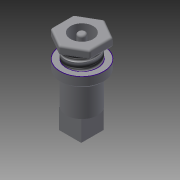
# Autodesk Inventor part: Power_Socket
Saved by Autodesk Inventor 2015 (Build 190159000, 159)
## iProperties
Created: 2014-12-09
Part Number: Power_Socket
Material: Generic
Document SubType Name: Modeling
Designer: Temp2
Density: 1 g/cm^3
Appearance: Default
Author: Temp2
Autodesk Inventor part; units mm, degrees
ref_plane "YZ Plane" through (0, 0, 0) normal (1, 0, 0) x (0, 1, 0)
ref_plane "XZ Plane" through (0, 0, 0) normal (0, 1, 0) x (-1, 0, 0)
ref_plane "XY Plane" through (0, 0, 0) normal (0, 0, 1) x (1, 0, 0)
sketch "Sketch1" plane through (0, 0, 0) normal (0, 0, 1) x (1, 0, 0)
  circle A0 centre (0, 0) radius 5.5
  circle A1 centre (0, 0) radius 1
  circle A2 centre (0, 0) radius 3.9688
  circle A3 centre (0, 0) radius 2.85
  dimension "d0" = 11
  dimension "d1" = 2
  dimension "d2" = 7.9375
  dimension "d3" = 5.7
  constraints: 4 centre point, 4 coincident
  measures "d0" diameter of A0
  measures "d1" diameter of A1
  measures "d2" diameter of A2
  measures "d3" diameter of A3
extrude "Extrusion1" add sketch "Sketch1" along normal blind 5.7 and the other way blind 10.4 contours A2
extrude "Extrusion2" add sketch "Sketch1" against normal blind 2.7 contours A0
extrude "Extrusion3" add sketch "Sketch1" along normal blind 5.7 contours A1
extrude "Extrusion4" add sketch "Sketch1" against normal blind 2.7 contours A1 | A2 | A3
sketch "Sketch2" plane through (0, 0, -10.4) normal (0, 0, -1) x (-1, 0, 0)
  circle A0 centre (0, 0) radius 3.9688 projected
  line L0 (2.8725, 2.7386) -> (-2.7241, 2.7386)
  line L1 (-2.7241, 2.7386) -> (-2.7241, -2.8862)
  line L2 (-2.7241, -2.8862) -> (2.8725, -2.8862)
  line L3 (2.8725, -2.8862) -> (2.8725, 2.7386)
  constraints: 8 end point, 2 parallel, 2 point on circle, 1 horizontal, 1 perpendicular
extrude "Extrusion5" add sketch "Sketch2" along normal blind 5.2 contours L3 A0 L2 L1 L0 | L3 L2 A0
sketch "Sketch3" plane through (0, 0, 5.7) normal (0, 0, 1) x (1, 0, 0)
  line L0 (5, -2.8868) -> (5, 2.8868)
  line L1 (0, 5.7735) -> (5, 2.8868)
  line L2 (0, 5.7735) -> (-5, 2.8868)
  line L3 (-5, 2.8868) -> (-5, -2.8868)
  line L4 (-5, -2.8868) -> (0, -5.7735)
  line L5 (0, -5.7735) -> (5, -2.8868)
  circle A0 centre (0, 0) radius 3.9688
  constraints: 12 end point, 3 parallel, 1 centre point, 1 coincident, 1 vertical
extrude "Extrusion6" add sketch "Sketch3" against normal blind 2.1
fillet "Fillet1" radius 0.5 18 edges at (-2.5, -4.3301, 5.7) (2.5, -4.3301, 5.7) (2.5, -4.3301, 3.6) (-2.5, -4.3301, 3.6) (-5, 0, 3.6) (-5, 0, 5.7) (5, 0, 5.7) (2.5, 4.3301, 5.7) (-2.5, 4.3301, 5.7) (0, -5.7735, 4.65) (5, -2.8868, 4.65) (-5, -2.8868, 4.65) (-5, 2.8868, 4.65) (-2.5, 4.3301, 3.6) (0, 5.7735, 4.65) (2.5, 4.3301, 3.6) (5, 2.8868, 4.65) (5, 0, 3.6)
fillet "Fillet2" radius 0.5 1 edges at (-1, 0, 5.7)
chamfer "Chamfer1" distance 0.5 angle 45 1 edges at (-5.5, 0, -2.7)
thread "Thread1" size "5/16-12" class "2B" standard "Inch Tapping Threads" length 15.255
body "Solid1"
